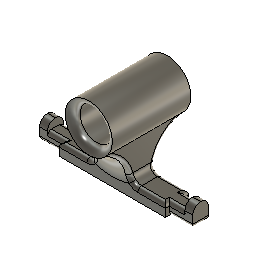
7-Attache_electronique (Autodesk Fusion 360 design; units mm, degrees)
Autodesk Fusion 360 part; units mm, degrees
sketch "Sketch1" plane through (0, 0, 0) normal (0, 0, 1) x (1, 0, 0)
  line L0 (-13.5, -3) -> (0, -3)
  line L1 (0, -3) -> (0, 0)
  line L2 (0, 0) -> (-13.5, 0)
  line L3 (-13.5, 0) -> (-13.5, -3)
  line L4 (-13.5, -0.5) -> (-15.5, -0.5)
  line L5 (-15.5, -0.5) -> (-15.5, -2.5)
  line L6 (-15.5, -2.5) -> (-13.5, -2.5)
  line L7 (-13.5, -2.5) -> (-13.5, -0.5)
  line L8 (0, -0.5) -> (2, -0.5)
  line L9 (2, -0.5) -> (2, -2.5)
  line L10 (2, -2.5) -> (0, -2.5)
  line L11 (0, -2.5) -> (0, -0.5)
  line L12 (-15.5, -0.5) -> (-16.5, -0.5)
  line L13 (-16.5, -0.5) -> (-16.5, -2.5)
  line L14 (-16.5, -2.5) -> (-15.5, -2.5)
  line L15 (-15.5, -2.5) -> (-15.5, -0.5)
  line L16 (2, -2.5) -> (3, -2.5)
  line L17 (3, -2.5) -> (3, -0.5)
  line L18 (3, -0.5) -> (2, -0.5)
  line L19 (2, -0.5) -> (2, -2.5)
  dimension "d1" = 13.5
  dimension "d2" = 3
  dimension "d3" = 2
  dimension "d4" = 2
  dimension "d5" = 0.5
  dimension "d6" = 2
  dimension "d7" = 2
  dimension "d8" = 0.5
  dimension "d11" = 1
  dimension "d12" = 2
  dimension "d13" = 1
  dimension "d14" = 2
  measures "d1" distance of L1 L3
  measures "d2" distance of L0 L2
  measures "d4" distance of L4 L6
  measures "d5" distance of L2 L4
  measures "d6" distance of L1 L9
  measures "d7" distance of L8 L10
  measures "d8" distance of L2 L8
  measures "d11" distance of L9 L17
  measures "d12" distance of L16 L18
  measures "d13" distance of L5 L13
  measures "d14" distance of L12 L14
extrude "Extrude2" add sketch "Sketch1" along normal blind 2.5 contours L5 L12 L13 L14 L15 | L9 L16 L17 L18 L19 makes body 1 at (-15.5, -1.1667, 0.8333) makes body 2 at (2, -1.1667, 0.8333)
extrude "Extrude1" add sketch "Sketch1" along normal blind 1.5 separate body contours L0 L1 L2 L3 L7 L11 | L3 L4 L5 L6 L7 L15 | L1 L8 L9 L10 L11 L19 makes body 3
fillet "Fillet1" radius 1 4 edges at (-16, -2.5, 2.5) (-16, -0.5, 2.5) (2.5, -0.5, 2.5) (2.5, -2.5, 2.5) on bodies 1 2
fillet "Fillet2" radius 0.5 10 edges at (-14.5, -2.5, 0) (1, -2.5, 0) (1, -0.5, 0) (-14.5, -0.5, 0) (-16, -2.5, 0) (-16, -0.5, 0) (-16.5, -1.5, 0) (2.5, -2.5, 0) (3, -1.5, 0) (2.5, -0.5, 0) on bodies 1 2 3
sketch "Sketch2" plane through (0, -3, 0) normal (0, -1, 0) x (1, 0, 0)
  line L0 (-13.5, 0) -> (0, 0)
  line L1 (0, 0) -> (0, 1.5)
  line L2 (0, 1.5) -> (-13.5, 1.5)
  line L3 (-13.5, 1.5) -> (-13.5, 0)
  circle A0 centre (-6.75, 8) radius 3
  line L4 (-13.5, 0) -> (0, 0)
  circle A1 centre (-6.75, 8) radius 2.1
  line L5 (-9, 7) -> (-4.5, 7)
  line L6 (-4.5, 7) -> (-4.5, 1.5)
  line L7 (-4.5, 1.5) -> (-9, 1.5)
  line L8 (-9, 1.5) -> (-9, 7)
  dimension "d19" = 6
  dimension "d20" = 8
  dimension "d21" = 6.75
  dimension "d22" = 4.2
  dimension "d32" = 4.5
  dimension "d33" = 5.5
  dimension "d34" = 2.25
  measures "d19" diameter of A0
  measures "d20" distance of L4
  measures "d21" distance of L0.end
  measures "d22" diameter of A1
  measures "d32" distance of L6 L8
  measures "d33" distance of L5 L7
  measures "d34" distance of L6
extrude "Extrude5" add sketch "Sketch2" against normal blind 3 contours L2 A0 L6 L7 L8 bodies 3
extrude "Extrude4" cut sketch "Sketch2" against normal blind 4 contours A1 L5 | A1 L5 bodies 3
extrude "Extrude3" add sketch "Sketch2" along normal blind 3 and the other way blind 7 contours A0 A1 L5 L6 L8 | A0 A1 L5 L6 L8 bodies 3
fillet "Fillet5" radius 1 2 edges at (-8.7079, 4, 7.2406) (-8.7079, -6, 8.7594) on bodies 3
combine "Combine1" operation add target body 1 tool bodies 2 3
fillet "Fillet6" radius 4 2 edges at (-6.75, -3, 5) (-6.75, 0, 5) on bodies 1
fillet "Fillet7" radius 1 2 edges at (-9, -1.4991, 1.5) (-4.5, -1.4991, 1.5) on bodies 1
fillet "Fillet8" radius 0.5 24 edges at (-14.5, -2.5, 1.5) (-13.5, -0.25, 1.5) (-14.5, -0.5, 1.5) (-9, 1.5264, 4.8653) (-9.1534, 0.0322, 1.9677) (-9.7819, 0, 1.5241) (-11.75, 0, 1.5) (-13.5, -2.75, 1.5) (-11.75, -3, 1.5) (-9.7052, -3, 1.5444) (-9.1145, -3.0262, 2.0353) (-9, -4.1468, 4.6088) (-4.5, -4.1468, 4.6088) (-4.3854, -3.0261, 2.0352) (-3.7948, -3, 1.5444) (-1.75, -3, 1.5) (0, -2.75, 1.5) (1, -2.5, 1.5) (0, -0.25, 1.5) (1, -0.5, 1.5) (-1.75, 0, 1.5) (-3.7181, 0, 1.5241) (-4.3466, 0.0322, 1.9677) (-4.5, 1.5264, 4.8653) on bodies 1
